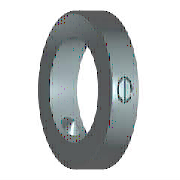
# Autodesk Inventor part: Unbrako. Hallowell Steel Collars. Inch Series - 0.5 x 1 x 7/16
Saved by Autodesk Inventor 2021 (Build 250183000, 183)
## iProperties
Created: 2020-01-21
Part Number: Unbrako. Hallowell Steel Collars. Inch Series - 0.5 x 1 x 7/16
Material: Acero, suave
Description: Anillo de ajuste
Document SubType Name: Modeling
Standard: Unbrako  (Collares de acero Hallowell. Serie en pulgadas)
Designer: 79449
Standards Organization: ANSI
Language: es-ES
Size Designation: 0.5 x 1 x 7/16
Categories: <MemberInstance><Categories><Category DisplayName="Piezas del eje" InternalName="7f7aeb1f-a693-4053-b835-cee3144e0d98" Mnemonic="SHFT"><Category DisplayName="Collares" InternalName="c4613f1d-9466-474f-9903-77ea01561514" Mnemonic="COLLAR"><CategoryParameter DisplayName="Anchura" InternalName="03f05fad-a492-4389-af6c-81edd2da50a5" Mnemonic="wdth"/><CategoryParameter DisplayName="Diámetro de eje" InternalName="6cfdf424-e5c2-4a0c-a45e-da080b42b5a6" Mnemonic="shaftdia"/><CategoryParameter DisplayName="Diámetro exterior" InternalName="f7e5b2bc-5a75-495b-a7c1-03452745573f" Mnemonic="outdia"/></Category></Category><Category DisplayName="TipoDatos" InternalName="23b78d0f-2648-40c6-8793-ca6db495c9e8" Mnemonic="DATATYPE"><CategoryParameter DisplayName="NombreVisualización" InternalName="05415f3d-3907-474b-a020-eb9d644f4cf3" Mnemonic="DISPLAYNAME"/><CategoryParameter DisplayName="Estándar" InternalName="0c0a119c-1e12-4c84-803f-101930972f5e" Mnemonic="STANDARD"/><CategoryParameter DisplayName="Descripción" InternalName="13903e3d-64b1-4950-80da-f627842ea37f" Mnemonic="DESCRIPTION"/><CategoryParameter DisplayName="Designación" InternalName="2675968c-4ce5-49e0-a4f5-552d29089031" Mnemonic="DESIGNATION"/><CategoryParameter DisplayName="Fila por defecto" InternalName="2af9ec52-faaa-4026-b378-f9fa4afca842" Mnemonic="DEFAULTROW"/><CategoryParameter DisplayName="Nombre de carpeta" InternalName="3f06958e-8713-4116-9be7-ed6184ecc97b" Mnemonic="FOLDERNAME"/><CategoryParameter DisplayName="Guid de revisión" InternalName="45a75005-10b1-4dfc-8d6d-dfe629f0b93c" Mnemonic="REVISIONGUID"/><CategoryParameter DisplayName="NombreArchivo" InternalName="8b46a4cc-9585-4fed-90c3-899f57e09a73" Mnemonic="FILENAME"/><CategoryParameter DisplayName="OrgEstand" InternalName="8f5914e1-4693-403f-8ab5-d37768198c9d" Mnemonic="STDSORG"/><CategoryParameter DisplayName="Versión de familia" InternalName="914462f6-6e19-4b14-ba84-155b9680b1d0" Mnemonic="FAMILYREVISION"/><CategoryParameter DisplayName="Revisión de Norma" InternalName="91d5a463-65c2-4fde-b823-3b7fea5e8e17" Mnemonic="STANDARDREVISION"/><CategoryParameter DisplayName="Revisión del miembro" InternalName="a65d44b9-392f-4f4f-857b-e4b3d54996fe" Mnemonic="MEMBERREVISION"/><CategoryParameter DisplayName="FormatoDelimitación" InternalName="bc51e27b-3422-4e78-93ef-cec197ddf230" Mnemonic="CLIPFORMAT"/><CategoryParameter DisplayName="Fabricante" InternalName="cd6c7a72-a28a-4e50-99a9-2c7f4e13e5ad" Mnemonic="MANUFACTURER"/><CategoryParameter DisplayName="NombreInterno" InternalName="cf1d0246-76d9-4b4a-8305-fa0409afb5c1" Mnemonic="INTERNALNAME"/><CategoryParameter DisplayName="EsMétrico" InternalName="e2385c5b-1ea4-4823-96a8-8de651266ec3" Mnemonic="ISMETRIC"/><Category DisplayName="Pieza" InternalName="c0e0b642-3bcb-4cc8-9e80-f96d35c4afa4" Mnemonic="PART"><CategoryParameter DisplayName="Número de pieza" InternalName="016b6077-bfbe-49bd-92c9-d8d59c39c941" Mnemonic="PARTNUMBER"/><CategoryParameter DisplayName="Referencia de almacén" InternalName="4dba7c1c-e26c-444e-836c-b08b433409a8" Mnemonic="STOCKNUMBER"/><CategoryParameter DisplayName="Clave de material" InternalName="5c9a8adb-dd2b-4535-b97f-0a94a95fe41f" Mnemonic="MATERIALKEY"/><CategoryParameter DisplayName="Material" InternalName="818a152a-d3c3-49ca-80ee-df7d91421b8e" Mnemonic="MATERIAL"/></Category></Category><Category DisplayName="AsignaciónHeredada" InternalName="cd87c42b-3e48-431e-b5c0-1cbeb14dfe77" Mnemonic="LEGACYMAP"><CategoryParameter DisplayName="Id de miembro DA exclusivo" InternalName="0918ad47-427f-4fed-ae26-24c81c58f590" Mnemonic="DACOOKIE"/><CategoryParameter DisplayName="Fusión11 ID" InternalName="0ee8fb18-e2ed-4f39-96f6-1f4b5f50aa71" Mnemonic="MERGE11"/><CategoryParameter DisplayName="Id. de miembro CC exclusivo" InternalName="5193edd4-b2b0-4ab4-9d54-de900eee34e0" Mnemonic="CCCOOKIE"/><CategoryParameter DisplayName="División ID" InternalName="72b5c83c-be7f-45c4-ae51-9160ea6deb26" Mnemonic="SPLIT"/><CategoryParameter DisplayName="IDMiembro" InternalName="8e5e0294-fc51-4c8f-b3d7-003dc5ed94f6" Mnemonic="MEMBERID"/><CategoryParameter DisplayName="NombreCatálogo" InternalName="d99d1e27-aa94-4de2-af4c-c348882a6f4f" Mnemonic="CATALOGNAME"/><CategoryParameter DisplayName="NúmeroFamilia" InternalName="e705e1f4-09cb-413e-91f9-551b4188271e" Mnemonic="FAMILYNUMBER"/></Category></Categories><FamilyTemplate Id="no0092"><FamilyTemplateParameters><FamilyTemplateParameter ObjectType="kUserParameterObject" ValueType="xs:double" Id="1" ObjectReferenceKey="WND"/><FamilyTemplateParameter ObjectType="kUserParameterObject" ValueType="xs:double" Id="2" ObjectReferenceKey="NND1"/><FamilyTemplateParameter ObjectType="kUserParameterObject" ValueType="xs:double" Id="3" ObjectReferenceKey="RR"/><FamilyTemplateParameter ObjectType="kUserParameterObject" ValueType="xs:double" Id="4" ObjectReferenceKey="GD1"/><FamilyTemplateParameter ObjectType="kUserParameterObject" ValueType="xs:double" Id="5" ObjectReferenceKey="SD2"/><FamilyTemplateParameter ObjectType="kUserParameterObject" ValueType="xs:double" Id="6" ObjectReferenceKey="PHH"/><FamilyTemplateParameter ObjectType="kUserParameterObject" ValueType="xs:double" Id="7" ObjectReferenceKey="SD"/><FamilyTemplateParameter ObjectType="kUserParameterObject" ValueType="xs:double" Id="8" ObjectReferenceKey="NND"/><FamilyTemplateParameter ObjectType="kUserParameterObject" ValueType="xs:double" Id="9" ObjectReferenceKey="FAWI"/><FamilyTemplateParameter ObjectType="kPropertyObject" ValueType="xs:string" Id="100" ObjectReferenceKey="{32853F0F-3444-11d1-9E93-0060B03C1CA6}" SubObjectId="52"/><FamilyTemplateParameter ObjectType="kPropertyObject" ValueType="xs:string" Id="105" ObjectReferenceKey="{32853F0F-3444-11d1-9E93-0060B03C1CA6}" SubObjectId="5"/><FamilyTemplateParameter ObjectType="kPartComponentDefinitionObject" ValueType="xs:string" Id="110" SubObjectId="Material"/></FamilyTemplateParameters></FamilyTemplate><CategoryParameterMap><ParamToTemplateMap><ParamToTemplate CategoryParameter="//CategoryParameter[@InternalName='05415f3d-3907-474b-a020-eb9d644f4cf3']" ConstantValue="Adjusting Ring"/><ParamToTemplate CategoryParameter="//CategoryParameter[@InternalName='cf1d0246-76d9-4b4a-8305-fa0409afb5c1']" ConstantValue="dd7bd0e9-b0fd-44c8-80d6-476c9181ebed"/><ParamToTemplate CategoryParameter="//CategoryParameter[@InternalName='3f06958e-8713-4116-9be7-ed6184ecc97b']" ConstantValue="U 3284(2)"/><ParamToTemplate CategoryParameter="//CategoryParameter[@InternalName='914462f6-6e19-4b14-ba84-155b9680b1d0']" ConstantValue="10"/><ParamToTemplate CategoryParameter="//CategoryParameter[@InternalName='bc51e27b-3422-4e78-93ef-cec197ddf230']" ConstantValue="CF_INVENTOR.STDPARTS"/><ParamToTemplate CategoryParameter="//CategoryParameter[@InternalName='e2385c5b-1ea4-4823-96a8-8de651266ec3']" ConstantValue="false"/><ParamToTemplate CategoryParameter="//CategoryParameter[@InternalName='13903e3d-64b1-4950-80da-f627842ea37f']" ConstantValue="Adjusting Ring"/><ParamToTemplate CategoryParameter="//CategoryParameter[@InternalName='8f5914e1-4693-403f-8ab5-d37768198c9d']" ConstantValue="ANSI"/><ParamToTemplate CategoryParameter="//CategoryParameter[@InternalName='0c0a119c-1e12-4c84-803f-101930972f5e']" ConstantValue="Unbrako  (Hallowell Steel Collars. Inch Series)"/><ParamToTemplate CategoryParameter="//CategoryParameter[@InternalName='cd6c7a72-a28a-4e50-99a9-2c7f4e13e5ad']" TemplateParameter="104"/><ParamToTemplate CategoryParameter="//CategoryParameter[@InternalName='91d5a463-65c2-4fde-b823-3b7fea5e8e17']" TemplateParameter="103"/><ParamToTemplate CategoryParameter="//CategoryParameter[@InternalName='45a75005-10b1-4dfc-8d6d-dfe629f0b93c']" ConstantValue="26fd7685-ed8e-4ce2-b2d6-33b3e992839e"/><ParamToTemplate CategoryParameter="//CategoryParameter[@InternalName='2af9ec52-faaa-4026-b378-f9fa4afca842']" ConstantValue="1"/><ParamToTemplate CategoryParameter="//CategoryParameter[@InternalName='d99d1e27-aa94-4de2-af4c-c348882a6f4f']" ConstantValue="ANSI"/><ParamToTemplate CategoryParameter="//CategoryParameter[@InternalName='e705e1f4-09cb-413e-91f9-551b4188271e']" ConstantValue="1257"/><ParamToTemplate CategoryParameter="//CategoryParameter[@InternalName='8b46a4cc-9585-4fed-90c3-899f57e09a73']" ConstantValue="Unbrako. Hallowell Steel Collars. Inch Series - 0.5 x 1 x 7/16"/><ParamToTemplate CategoryParameter="//CategoryParameter[@InternalName='a65d44b9-392f-4f4f-857b-e4b3d54996fe']" ConstantValue="19c5a0d7-8e45-4c80-9f41-3cb5cf71df8d"/><ParamToTemplate CategoryParameter="//CategoryParameter[@InternalName='8e5e0294-fc51-4c8f-b3d7-003dc5ed94f6']" ConstantValue="6"/><ParamToTemplate CategoryParameter="//CategoryParameter[@InternalName='2675968c-4ce5-49e0-a4f5-552d29089031']" TemplateParameter="100"/><ParamToTemplate CategoryParameter="//CategoryParameter[@InternalName='818a152a-d3c3-49ca-80ee-df7d91421b8e']" TemplateParameter="110"/><ParamToTemplate CategoryParameter="//CategoryParameter[@InternalName='016b6077-bfbe-49bd-92c9-d8d59c39c941']" TemplateParameter="105"/><ParamToTemplate CategoryParameter="//CategoryParameter[@InternalName='03f05fad-a492-4389-af6c-81edd2da50a5']" TemplateParameter="7"/><ParamToTemplate CategoryParameter="//CategoryParameter[@InternalName='f7e5b2bc-5a75-495b-a7c1-03452745573f']" TemplateParameter="5"/><ParamToTemplate CategoryParameter="//CategoryParameter[@InternalName='6cfdf424-e5c2-4a0c-a45e-da080b42b5a6']" TemplateParameter="1"/></ParamToTemplateMap></CategoryParameterMap></MemberInstance>
Density: 7.85 g/cm^3
Appearance: Semipulido
IsCustomPart: 0
Author: 79449
Autodesk Inventor part; units mm, degrees
ref_plane "YZ Plane" through (0, 0, 0) normal (1, 0, 0) x (0, 1, 0)
sketch "Boceto1" plane through (0, 0, 0) normal (0, 0, 1) x (1, 0, 0)
  line L0 (0, 12.7) -> (11.1125, 12.7)
  line L1 (-1.9497, 0) -> (21.5466, 0)
  line L2 (0, 12.7) -> (0, 6.35)
  line L3 (0, 6.35) -> (11.1125, 6.35)
  line L4 (11.1125, 6.35) -> (11.1125, 12.7)
  line L5 (-6.6489, 0) -> (26.2458, 0) projected
  line L6 (0, 54) -> (0, -9) projected
  dimension "d0" = 25.4
  dimension "d1" = 12.7
  dimension "d2" = 11.1125
  constraints: 10 end point, 2 perpendicular, 1 horizontal, 1 parallel, 1 vertical
  measures "d0" diameter of L0 L1
  measures "d1" diameter of L3 L1
  measures "d2" distance between parallel lines of L4 L2
revolve "Cuerpo" add sketch "Boceto1" angle 360 about axis through (-1.9497, 0, 0) along (1, 0, 0)
ref_plane "IDS_WORKPLANE{1}" through (0, 12.7, 0) normal (0, 1, 0) x (-1, 0, 0)
sketch "Boceto2" plane through (0, 12.7, 0) normal (0, 1, 0) x (-1, 0, 0)
  line L0 (0, 12.7) -> (0, -12.7) projected
  line L1 (-12.156, 0) -> (2.026, 0) projected
  point P0 (-5.5563, 0)
  dimension "d7" = 5.5563
  constraints: 1 point on line
  measures "d7" distance from line of L0 point (-5.556, 0)
hole "Agujero1" at (5.5563, 12.7, 0) direction (0, -1, 0) diameter 6.35 depth 12.7 tip angle 118
ref_plane "IDS_WORKPLANE{2}" through (5.5563, 0, 0) normal (-1, 0, 0) x (0, 0, 1)
sketch "Boceto3" plane through (5.5563, 0, 0) normal (-1, 0, 0) x (0, 0, 1)
  line L0 (0, 12.7) -> (1.7831, 12.7)
  line L1 (1.7831, 12.7) -> (3.175, 12.4041)
  line L2 (3.175, 12.4041) -> (3.175, 7.1157)
  line L3 (0, 56.54) -> (0, -24.24) projected
  circle A0 centre (0, 0) radius 12.7 projected
  line L4 (0, 12.7) -> (0, 6.35)
  line L5 (3.175, 7.1157) -> (0.3175, 6.35)
  line L6 (0.3175, 6.35) -> (0, 6.35)
  dimension "d18" = 3.5662
  dimension "d19" = 6.35
  dimension "d20" = 0.635
  dimension "d21" = 6.35
  dimension "d30" = 15
  dimension "d31" = 12
  constraints: 12 end point, 2 perpendicular, 2 point on line, 1 collinear, 1 horizontal, 1 horizontal alignment, 1 tangent
  measures "d18" diameter of L0.end L4
  measures "d19" diameter of L2 L4
  measures "d20" diameter of L5.end L4
  measures "d21" distance between parallel lines of L0 L6
  measures "d30" angle of L6 L5
  measures "d31" angle of L1 L0
revolve "Tornillo de cabeza perdida1" add sketch "Boceto3" angle 360 about axis through (5.5563, 12.7, 0) along (0, -1, 0) picked at (1.5203, 8.7069) contours A0 L2 L5 L6 L3 | L0 L1 L2 A0
sketch "Boceto4" plane through (0, 12.7, 0) normal (0, 1, 0) x (-1, 0, 0)
  line L0 (-5.5562, 1.27) -> (-4.4564, 0.635)
  line L1 (-4.4564, 0.635) -> (-4.4564, -0.635)
  line L2 (-4.4564, -0.635) -> (-5.5563, -1.27)
  line L3 (-5.5563, -1.27) -> (-6.6561, -0.635)
  line L4 (-6.6561, -0.635) -> (-6.6561, 0.635)
  line L5 (-6.6561, 0.635) -> (-5.5562, 1.27)
  line L6 (-14.2345, 0) -> (2.3724, 0) projected
  line L7 (0, 6.35) -> (0, -6.35) projected
  point P0 (-5.5563, 0)
  dimension "d22" = 2.54
  dimension "d23" = 5.5563
  constraints: 12 end point, 1 point on line, 1 vertical, 11 other
  measures "d22" distance of L0.start L2.end
  measures "d23" distance from line of L7 point (-5.556, 0)
extrude "Ranura1" cut sketch "Boceto4" against normal blind 1.5875
chamfer "Chaflán1" distance 1.1112 angle 15 1 edges at (11.1125, -12.7, 0) measured on face at (3.7042, 10.7339, 6.7877)
chamfer "Chaflán2" distance 0.1905 distance2 1.1112 1 edges at (11.1125, -6.35, 0) measured on face at (11.1125, 10.2032, -1.4959)
fillet "Empalme1" radius 0.5558 1 edges at (0, -12.7, 0)
equation "\"d7\" = 0.5 * SD"
equation "\"d18\" = GD1"
equation "\"d19\" = NND"
equation "\"d20\" = 0.1 * NND"
equation "\"d21\" = -0.5 * WND + 0.5 * SD2"
equation "\"d30\" = FAWI"
equation "\"d31\" = 0.8 * FAWI"
equation "\"d22\" = 0.4 * NND"
equation "\"d23\" = 0.5 * SD"
equation "\"d24\" = 0.25 * NND"
equation "\"d8\" = NND"
equation "\"d13\" = 0.5 * SD2"
equation "\"d4\" = PHH"
equation "\"d5\" = FAWI"
equation "\"d59\" = PHH"
equation "\"d26\" = -0.5 * WND + 0.5 * NND1"
equation "\"d27\" = PHH"
equation "\"d29\" = RR"
equation "\"d0\" = SD2"
equation "\"d1\" = WND"
equation "\"d2\" = SD"
equation "\"WND\" = 12.7"
equation "\"SD2\" = 25.4"
equation "\"SD\" = 11.1125"
equation "\"NND\" = 6.35"
equation "\"FAWI\" = 15deg"
equation "\"PHH\" = 1.11125"
equation "\"d6\" = 0.5 * SD2"
equation "\"GD1\" = 3.56616"
equation "\"d17\" = -0.5 * SD"
equation "\"RR\" = 0.55575"
equation "\"NND1\" = 13.081"
body "Solid1"
